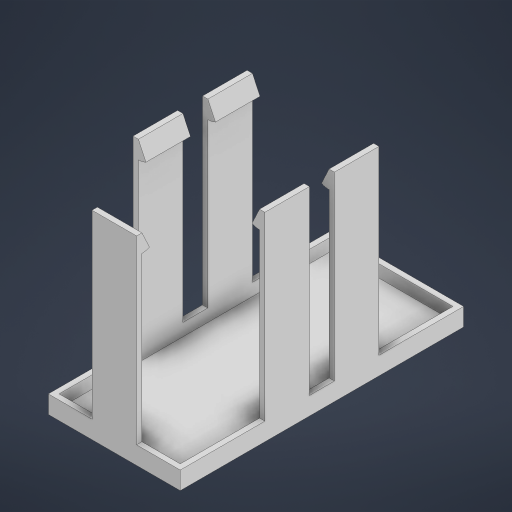
# Autodesk Inventor part: battery pack holder
Saved by Autodesk Inventor 2023 (Build 270158000, 158)
## iProperties
Created: 2022-09-20
Part Number: battery pack holder
Material: Generic
Document SubType Name: Modeling
Designer: CB110-09
Density: 1 g/cm^3
Appearance: Default
Author: CB110-09
Autodesk Inventor part; units mm, degrees
ref_plane "YZ Plane" through (0, 0, 0) normal (1, 0, 0) x (0, 1, 0)
ref_plane "XZ Plane" through (0, 0, 0) normal (0, 1, 0) x (-1, 0, 0)
ref_plane "XY Plane" through (0, 0, 0) normal (0, 0, 1) x (1, 0, 0)
sketch "Sketch1" plane through (0, 0, 0) normal (0, 1, 0) x (-1, 0, 0)
  line L0 (-37, -79.5) -> (37, -79.5)
  line L1 (37, -79.5) -> (37, 79.5)
  line L2 (37, 79.5) -> (-37, 79.5)
  line L3 (-37, 79.5) -> (-37, -79.5)
  line L4 (-37, -79.5) -> (37, 79.5) construction
  line L5 (37, -79.5) -> (-37, 79.5) construction
  point P0 (0, 0)
  dimension "d0" = 74
  dimension "d1" = 159
  constraints: 12 end point, 2 midpoint, 2 parallel, 1 horizontal, 1 perpendicular
  measures "d0" distance of L2.end L1.end
  measures "d1" distance of L1.end L0.end
extrude "Extrusion1" add sketch "Sketch1" along normal blind 3
sketch "Sketch2" plane through (0, 3, 0) normal (0, 1, 0) x (1, 0, 0)
  line L0 (34, 76.5) -> (-34, 76.5)
  line L1 (-34, 76.5) -> (-34, -76.5)
  line L2 (-34, -76.5) -> (34, -76.5)
  line L3 (34, -76.5) -> (34, 76.5)
  line L4 (34, 76.5) -> (-34, -76.5) construction
  line L5 (-34, 76.5) -> (34, -76.5) construction
  line L6 (-37, 79.5) -> (-37, -79.5) projected
  line L7 (-37, -79.5) -> (37, -79.5) projected
  line L8 (34, 7) -> (37, 7)
  line L9 (34, -7) -> (37, -7)
  line L10 (37, -79.5) -> (37, 79.5) projected
  line L11 (34, 32) -> (37, 32)
  line L12 (34, -32) -> (37, -32)
  line L13 (0, 0) -> (0, 8.1012)
  line L14 (-34, 7) -> (-37, 7)
  line L15 (-34, -7) -> (-37, -7)
  line L16 (-34, 32) -> (-37, 32)
  line L17 (-34, -32) -> (-37, -32)
  line L18 (-12.5, -79.5) -> (-12.5, -76.5)
  line L19 (12.5, -76.5) -> (12.5, -79.5)
  line L20 (-34, -32) -> (-34, -7)
  line L21 (-34, 7) -> (-34, -7)
  line L22 (-34, 32) -> (-34, 7)
  line L23 (-37, 7) -> (-37, 32)
  line L24 (-37, -7) -> (-37, -32)
  line L25 (34, -32) -> (34, -7)
  line L26 (37, -7) -> (37, -32)
  line L27 (34, 7) -> (34, 32)
  line L28 (37, 32) -> (37, 7)
  line L29 (12.5, -76.5) -> (-12.5, -76.5)
  line L30 (-12.5, -79.5) -> (12.5, -79.5)
  point P0 (35.5, -7)
  point P1 (34, 0)
  point P2 (35.5, 7)
  point P3 (35.5, 32)
  point P4 (35.5, -32)
  point P5 (0, -76.5)
  point P6 (12.5, -78)
  point P7 (-12.5, -78)
  dimension "d4" = 3
  dimension "d5" = 3
  dimension "d6" = 7
  dimension "d7" = 7
  dimension "d8" = 32
  dimension "d9" = 32
  dimension "d10" = 12.5
  dimension "d11" = 12.5
  constraints: 56 end point, 11 point on line, 10 midpoint, 9 collinear, 8 symmetric about line, 6 parallel, 3 horizontal, 2 perpendicular, 2 vertical
  measures "d4" distance between parallel lines of L6 L1
  measures "d5" distance between parallel lines of L7 L2
  measures "d6" vertical distance of point (35.5, -7) point (34, 0)
  measures "d7" vertical distance of point (35.5, 7) point (34, 0)
  measures "d8" vertical distance of point (34, 0) point (35.5, 32)
  measures "d9" vertical distance of point (35.5, -32) point (34, 0)
  measures "d10" horizontal distance of point (0, -76.5) point (12.5, -78)
  measures "d11" horizontal distance of point (0, -76.5) point (-12.5, -78)
extrude "Extrusion2" add sketch "Sketch2" along normal blind 108.5 contours L11 L10 L8 L3 | L1 L14 L6 L16 | L9 L10 L12 L3 | L1 L17 L6 L15 | L19 L7 L18 L2
sketch "Sketch3" plane through (-34, 3, 32) normal (1, 0, 0) x (0, 0, -1)
  line L0 (25, 108.5) -> (0, 108.5) projected
  line L1 (0, 108.5) -> (25, 108.5)
  line L2 (25, 108.5) -> (25, 98.5)
  line L3 (25, 98.5) -> (0, 98.5)
  line L4 (0, 98.5) -> (0, 108.5)
  line L5 (39, 0) -> (39, 108.5) projected
  line L6 (39, 108.5) -> (64, 108.5)
  line L7 (64, 108.5) -> (64, 98.5)
  line L8 (64, 98.5) -> (39, 98.5)
  line L9 (39, 98.5) -> (39, 108.5)
  point P0 (32, -3)
  dimension "d14" = 25
  dimension "d15" = 10
  dimension "d16" = 25
  dimension "d17" = 10
  constraints: 16 end point, 4 parallel, 2 horizontal, 2 perpendicular
  measures "d14" distance of L2.end L3.end
  measures "d15" distance of L1.end L2.end
  measures "d16" distance of L7.end L8.end
  measures "d17" distance of L6.end L7.end
sketch "Sketch4" plane through (12.5, 3, 76.5) normal (0, 0, -1) x (-1, 0, 0)
  line L0 (0, 108.5) -> (25, 108.5) projected
  line L1 (0, 108.5) -> (25, 108.5)
  line L2 (25, 108.5) -> (25, 98.5)
  line L3 (25, 98.5) -> (0, 98.5)
  line L4 (0, 98.5) -> (0, 108.5)
  point P0 (12.5, -3)
  dimension "d18" = 25
  dimension "d19" = 10
  constraints: 8 end point, 2 parallel, 1 horizontal, 1 perpendicular
  measures "d18" distance of L2.end L3.end
  measures "d19" distance of L1.end L2.end
sketch "Sketch5" plane through (34, 3, 7) normal (-1, 0, 0) x (0, 0, 1)
  line L0 (-14, 108.5) -> (-39, 108.5) projected
  line L1 (-39, 108.5) -> (-14, 108.5)
  line L2 (-14, 108.5) -> (-14, 98.5)
  line L3 (-14, 98.5) -> (-39, 98.5)
  line L4 (-39, 98.5) -> (-39, 108.5)
  line L5 (0, 108.5) -> (25, 108.5)
  line L6 (25, 108.5) -> (25, 98.5)
  line L7 (25, 98.5) -> (0, 98.5)
  line L8 (0, 98.5) -> (0, 108.5)
  point P0 (-7, -3)
  dimension "d20" = 25
  dimension "d21" = 10
  dimension "d22" = 25
  dimension "d23" = 10
  constraints: 16 end point, 4 parallel, 2 horizontal, 2 perpendicular
  measures "d20" distance of L2.end L3.end
  measures "d21" distance of L1.end L2.end
  measures "d22" distance of L6.end L7.end
  measures "d23" distance of L5.end L6.end
revolve "Revolution1" add sketch "Sketch5" angle 25 about axis through (34, 111.5, 7) along (0, 0, -1)
revolve "Revolution2" add sketch "Sketch4" angle 25 about axis through (12.5, 111.5, 76.5) along (1, 0, 0)
revolve "Revolution3" add sketch "Sketch3" angle 25 about axis through (-34, 111.5, 7) along (0, 0, 1)
sketch "Sketch6" plane through (0, 3, 0) normal (0, 1, 0) x (1, 0, 0)
  line L0 (34, -76.5) -> (-34, -76.5)
  line L1 (-34, -76.5) -> (-34, 76.5)
  line L2 (-34, 76.5) -> (34, 76.5)
  line L3 (34, 76.5) -> (34, -76.5)
  line L4 (12.5, -79.5) -> (37, -79.5) projected
  line L5 (37, -79.5) -> (37, -32) projected
  line L6 (-37, -32) -> (-37, -79.5) projected
  line L7 (37, 79.5) -> (-37, 79.5) projected
  line L8 (-37, 79.5) -> (-37, -79.5) projected
  line L9 (37, -79.5) -> (-37, -79.5)
  line L10 (-37, -79.5) -> (-37, 79.5)
  line L11 (-37, 79.5) -> (37, 79.5)
  line L12 (37, 79.5) -> (37, -79.5)
  point P0 (0, 0)
  dimension "d27" = 3
  dimension "d28" = 3
  dimension "d29" = 3
  dimension "d30" = 3
  constraints: 16 end point, 4 parallel, 2 horizontal, 2 perpendicular
  measures "d27" distance between parallel lines of L4 L0
  measures "d28" distance between parallel lines of L5 L3
  measures "d29" distance between parallel lines of L6 L1
  measures "d30" distance between parallel lines of L7 L2
extrude "Extrusion3" add sketch "Sketch6" along normal blind 7
body "Solid1"
